Autodesk Fusion 360 part; units mm, degrees
(part 2 of 2)
  dimension "d115" = 6
  dimension "d116" = 6
  dimension "d117" = 6
  dimension "d118" = 6
  dimension "d119" = 6
  dimension "d120" = 6
  dimension "d121" = 6
  dimension "d122" = 6
  dimension "d123" = 6
  dimension "d124" = 6
  dimension "d125" = 6
  dimension "d126" = 6
  dimension "d195" = 0
  dimension "d196" = 40
  dimension "d199" = 0
  dimension "d200" = -133.5
  dimension "d203" = 240
  dimension "d204" = 0
  dimension "d207" = 0
  dimension "d208" = -240
  dimension "d211" = 0
  dimension "d212" = -133
  dimension "d215" = 0
  dimension "d216" = 40
  dimension "d219" = 0
  dimension "d220" = -269.838
  dimension "d223" = 0
  dimension "d224" = 269.838
  dimension "d225" = 200
  dimension "d226" = 330
  dimension "d227" = 40
  dimension "d228" = 40
  dimension "d229" = 40
  dimension "d230" = 40
  dimension "d231" = 60
  dimension "d232" = 90
  dimension "d233" = 90
  dimension "d234" = 110
  dimension "d235" = 110
  dimension "d236" = 110
  dimension "d237" = 120
  dimension "d238" = 55
  dimension "d239" = 55
  dimension "d240" = 55
  dimension "d241" = 55
  dimension "d242" = 16
  dimension "d243" = 25
  dimension "d244" = 25
  dimension "d245" = 35
  dimension "d246" = 12
  dimension "d247" = 19
  dimension "d248" = 50
  dimension "d249" = 5
  dimension "d250" = 150
  dimension "d251" = 22
  dimension "d252" = 22.5
  dimension "d253" = 22
  dimension "d254" = 6
  dimension "d255" = 200
  dimension "d256" = 269.3626
  dimension "d257" = 22
  dimension "d258" = 30
  dimension "d259" = 30
  dimension "d260" = 6
  dimension "d261" = 330
  dimension "d262" = 30
  dimension "d263" = 6
  dimension "d264" = 30
  dimension "d265" = 6
  dimension "d266" = 30
  dimension "d267" = 6
  dimension "d268" = 30
  dimension "d269" = 6
  dimension "d270" = 30
  dimension "d271" = 6
  dimension "d272" = 30
  dimension "d273" = 6
  dimension "d274" = 30
  dimension "d275" = 6
  dimension "d276" = 60
  dimension "d277" = 6
  dimension "d278" = 40
  dimension "d279" = 60
  dimension "d280" = 6
  dimension "d281" = 40
  dimension "d282" = 185.187
  dimension "d283" = 330
  dimension "d284" = 30
  dimension "d285" = 35
  dimension "d286" = 6
  dimension "d287" = 30
  dimension "d288" = 35
  dimension "d289" = 6
  dimension "d290" = 185.1872
  dimension "d291" = 185.187
  dimension "d292" = 30
  dimension "d293" = 30
  dimension "d294" = 6
  dimension "d295" = 35
  dimension "d296" = 15
  dimension "d297" = 10
  dimension "d298" = 6
  dimension "d299" = 35
  dimension "d300" = 330
  dimension "d301" = 20
  dimension "d302" = 17.5
  dimension "d303" = 6
  dimension "d304" = 6
  dimension "d305" = 6
  dimension "d306" = 6
  dimension "d307" = 6
  dimension "d308" = 6
  dimension "d309" = 6
  dimension "d310" = 6
  dimension "d311" = 6
  dimension "d312" = 6
  dimension "d313" = 6
  dimension "d314" = 6
  dimension "d315" = 6
  dimension "d316" = 6
  dimension "d317" = 6
  dimension "d318" = 6
  dimension "d319" = 6
  dimension "d320" = 6
  dimension "d321" = 6
  dimension "d322" = 6
  dimension "d323" = 6
  dimension "d324" = 6
  dimension "d325" = 6
  dimension "d326" = 6
  dimension "d327" = 6
  dimension "d328" = 6
  dimension "d329" = 6
  dimension "d330" = 6
  dimension "d331" = 300
  dimension "d332" = 35
  dimension "d333" = 5
  dimension "d334" = 150
  dimension "d335" = 20
  dimension "d336" = 200
  dimension "d337" = 269.3626
  dimension "d338" = 22
  dimension "d339" = 60
  dimension "d340" = 6
  dimension "d341" = 40
  dimension "d342" = 60
  dimension "d343" = 6
  dimension "d344" = 40
  dimension "d345" = 30
  dimension "d346" = 35
  dimension "d347" = 6
  dimension "d348" = 30
  dimension "d349" = 35
  dimension "d350" = 6
  dimension "d351" = 185.1872
  dimension "d352" = 35
  dimension "d353" = 15
  dimension "d354" = 10
  dimension "d355" = 6
  dimension "d356" = 6
  dimension "d357" = 6
  dimension "d358" = 6
  dimension "d359" = 6
  dimension "d360" = 6
  dimension "d361" = 6
  dimension "d362" = 6
  dimension "d363" = 6
  dimension "d364" = 6
  dimension "d365" = 6
  dimension "d366" = 6
  dimension "d367" = 5
  dimension "d368" = 20
  dimension "d369" = 5
  dimension "d370" = 6
  dimension "d371" = 5
  dimension "d372" = 9
  dimension "d373" = 20
  dimension "d374" = 9
  dimension "d375" = 5
  dimension "d376" = 9
  dimension "d377" = 9
  dimension "d378" = 9
  dimension "d379" = 9
  dimension "d380" = 9
  dimension "d381" = 9
  dimension "d382" = 9
  dimension "d383" = 9
  dimension "d384" = 9
  dimension "d385" = 9
  dimension "d386" = 9
  dimension "d387" = 6
  dimension "d388" = 15
  dimension "d389" = 6
  dimension "d390" = 15
  dimension "d391" = 6
  dimension "d392" = 15
  dimension "d393" = 6
  dimension "d394" = 15
  dimension "d395" = 6
  dimension "d396" = 15
  dimension "d397" = 6
  dimension "d398" = 15
  dimension "d399" = 6
  dimension "d400" = 5
  dimension "d401" = 9
  dimension "d402" = 20
  dimension "d403" = 9
  dimension "d404" = 5
  dimension "d405" = 6
  dimension "d406" = 6
  dimension "d407" = 5
  dimension "d408" = 9
  dimension "d409" = 20
  dimension "d410" = 9
  dimension "d411" = 5
  constraint vertical L19
  constraint horizontal L13
  constraint vertical L5
  constraint coincident L5.end L18.start
  constraint coincident L53.end L18
  constraint coincident L59.start L18
  constraint coincident L0.start L5
  constraint perpendicular L0 L5
  constraint horizontal L16
  constraint horizontal L11
  constraint horizontal L17
  constraint perpendicular L19 L56
  constraint perpendicular L19 L22
  constraint perpendicular L21 L56
  constraint perpendicular L19 L28
  constraint perpendicular L19 L61
  constraint perpendicular L24 L61
  constraint perpendicular L19 L20
  constraint perpendicular L19 L54
  constraint perpendicular L20 L52
  constraint perpendicular L27 L56
  constraint perpendicular L19 L30
  constraint perpendicular L18 L59
  constraint perpendicular L18 L23
  constraint perpendicular L18 L60
  constraint perpendicular L18 L36
  constraint perpendicular L14 L18
  constraint perpendicular L18 L42
  constraint perpendicular L18 L35
  constraint perpendicular L18 L39
  constraint perpendicular L18 L46
  constraint perpendicular L6 L18
  constraint perpendicular L5 L45
  constraint perpendicular L4 L5
  constraint perpendicular L4 L43
  constraint perpendicular L5 L51
  constraint perpendicular L5 L47
  constraint perpendicular L5 L37
  constraint horizontal L3
  constraint perpendicular L3 L8
  constraint perpendicular L11 L34
  constraint perpendicular L9 L11
  constraint perpendicular L31 L34
  constraint perpendicular L17 L32
  constraint perpendicular L1 L17
  constraint perpendicular L7 L32
  constraint perpendicular L11 L44
  constraint perpendicular L17 L48
  constraint perpendicular L44 L49
  constraint perpendicular L10 L13
  constraint perpendicular L11 L55
  constraint perpendicular L10 L15
  constraint perpendicular L17 L40
  constraint perpendicular L17 L25
  constraint perpendicular L40 L50
  constraint perpendicular L16 L58
  constraint perpendicular L17 L29
  constraint perpendicular L26 L58
  constraint vertical L81
  constraint horizontal L75
  constraint vertical L67
  constraint coincident L53.end L80
  constraint coincident L59.start L80
  constraint coincident L0.start L67
  constraint perpendicular L62 L67
  constraint horizontal L78
  constraint horizontal L73
  constraint horizontal L79
  constraint perpendicular L81 L118
  constraint perpendicular L81 L84
  constraint perpendicular L83 L118
  constraint perpendicular L81 L90
  constraint perpendicular L81 L123
  constraint perpendicular L86 L123
  constraint perpendicular L81 L82
  constraint perpendicular L81 L116
  constraint perpendicular L82 L114
  constraint perpendicular L89 L118
  constraint perpendicular L81 L92
  constraint perpendicular L80 L121
  constraint perpendicular L80 L85
  constraint perpendicular L80 L122
  constraint perpendicular L80 L98
  constraint perpendicular L76 L80
  constraint perpendicular L80 L104
  constraint perpendicular L80 L97
  constraint perpendicular L80 L101
  constraint perpendicular L80 L108
  constraint perpendicular L68 L80
  constraint perpendicular L67 L107
  constraint perpendicular L66 L67
  constraint perpendicular L66 L105
  constraint perpendicular L67 L113
  constraint perpendicular L67 L109
  constraint perpendicular L67 L99
  constraint horizontal L65
  constraint perpendicular L65 L70
  constraint perpendicular L73 L96
  constraint perpendicular L71 L73
  constraint perpendicular L93 L96
  constraint perpendicular L79 L94
  constraint perpendicular L63 L79
  constraint perpendicular L69 L94
  constraint perpendicular L73 L106
  constraint perpendicular L79 L110
  constraint perpendicular L106 L111
  constraint perpendicular L72 L75
  constraint perpendicular L73 L117
  constraint perpendicular L72 L77
  constraint perpendicular L79 L102
  constraint perpendicular L79 L87
  constraint perpendicular L102 L112
  constraint perpendicular L78 L120
  constraint perpendicular L79 L91
  constraint perpendicular L88 L120
  constraint vertical L143
  constraint horizontal L137
  constraint vertical L129
  constraint coincident L53.end L142
  constraint coincident L59.start L142
  constraint coincident L0.start L129
  constraint perpendicular L124 L129
  constraint horizontal L140
  constraint horizontal L135
  constraint horizontal L141
  constraint perpendicular L143 L180
  constraint perpendicular L143 L146
  constraint perpendicular L145 L180
  constraint perpendicular L143 L152
  constraint perpendicular L143 L185
  constraint perpendicular L148 L185
  constraint perpendicular L143 L144
  constraint perpendicular L143 L178
  constraint perpendicular L144 L176
  constraint perpendicular L151 L180
  constraint perpendicular L143 L154
  constraint perpendicular L142 L183
  constraint perpendicular L142 L147
  constraint perpendicular L142 L184
  constraint perpendicular L142 L160
  constraint perpendicular L138 L142
  constraint perpendicular L142 L166
  constraint perpendicular L142 L159
  constraint perpendicular L142 L163
  constraint perpendicular L142 L170
  constraint perpendicular L130 L142
  constraint perpendicular L129 L169
  constraint perpendicular L128 L129
  constraint perpendicular L128 L167
  constraint perpendicular L129 L175
  constraint perpendicular L129 L171
  constraint perpendicular L129 L161
  constraint horizontal L127
  constraint perpendicular L127 L132
  constraint perpendicular L135 L158
  constraint perpendicular L133 L135
  constraint perpendicular L155 L158
  constraint perpendicular L141 L156
  constraint perpendicular L125 L141
  constraint perpendicular L131 L156
  constraint perpendicular L135 L168
  constraint perpendicular L141 L172
  constraint perpendicular L168 L173
  constraint perpendicular L134 L137
  constraint perpendicular L135 L179
  constraint perpendicular L134 L139
  constraint perpendicular L141 L164
  constraint perpendicular L141 L149
  constraint perpendicular L164 L174
  constraint perpendicular L140 L182
  constraint perpendicular L141 L153
  constraint perpendicular L150 L182
  constraint perpendicular L315 L588
  constraint horizontal L348
  constraint vertical L466
  constraint perpendicular L190 L499
  constraint horizontal L231
  constraint vertical L386
  constraint horizontal L197
  constraint vertical L551
  constraint horizontal L337
  constraint vertical L254
  constraint horizontal L366
  constraint vertical L585
  constraint coincident L240.end L564
  constraint coincident L204.start L564
  constraint perpendicular L204 L564
  constraint perpendicular L204 L281
  constraint coincident L205.end L564
  constraint perpendicular L205 L564
  constraint coincident L528.start L588
  constraint coincident L568.start L588
  constraint coincident L583.end L588
  constraint coincident L548.start L588
  constraint coincident L343.start L588
  constraint coincident L339.start L588
  constraint coincident L372.start L588
  constraint coincident L325.start L588
  constraint coincident L558.start L588
  constraint coincident L305.start L523
  constraint perpendicular L523 L541
  constraint perpendicular L296 L541
  constraint coincident P228 L523
  constraint perpendicular L358 L523
  constraint coincident L305.start L360
  constraint perpendicular L333 L360
  constraint perpendicular L333 L335
  constraint coincident P228 L360
  constraint perpendicular L360 L538
  constraint perpendicular L304 L553
  constraint perpendicular L347 L351
  constraint perpendicular L341 L580
  constraint perpendicular L305 L342
  constraint perpendicular L572 L576
  constraint perpendicular L376 L595
  constraint coincident L293.start L315
  constraint perpendicular L293 L315
  constraint perpendicular L293 L329
  constraint coincident L357.end L315
  constraint perpendicular L315 L357
  constraint coincident L569.start L315
  constraint perpendicular L315 L569
  constraint perpendicular L525 L569
  constraint coincident L350.end L315
  constraint perpendicular L315 L350
  constraint horizontal L447
  constraint horizontal L330
  constraint vertical L298
  constraint coincident L533.start L540
  constraint perpendicular L533 L540
  constraint perpendicular L364 L533
  constraint coincident L290.end L540
  constraint perpendicular L290 L540
  constraint perpendicular L314 L540
  constraint perpendicular L314 L584
  constraint coincident L375.end L540
  constraint coincident L612.start L447
  constraint coincident L322.start L447
  constraint horizontal L459
  constraint coincident L291.start L459
  constraint coincident L300.start L459
  constraint coincident L319.start L298
  constraint perpendicular L298 L319
  constraint perpendicular L308 L319
  constraint coincident P107 L298
  constraint perpendicular L298 L332
  constraint coincident L556.start L190
  constraint perpendicular L190 L556
  constraint perpendicular L246 L556
  constraint coincident L409.end L190
  constraint perpendicular L190 L409
  constraint vertical L475
  constraint horizontal L486
  constraint vertical L509
  constraint coincident L314.start L498
  constraint coincident L227.start L250
  constraint coincident L384.start L250
  constraint coincident L251.start L486
  constraint coincident L429.start L486
  constraint perpendicular L558 L588
  constraint perpendicular L318 L588
  constraint perpendicular L372 L588
  constraint perpendicular L339 L588
  constraint perpendicular L343 L588
  constraint perpendicular L548 L588
  constraint perpendicular L568 L588
  constraint perpendicular L528 L588
  constraint perpendicular L369 L588
  constraint perpendicular L289 L459
  constraint perpendicular L291 L459
  constraint perpendicular L300 L447
  constraint perpendicular L322 L447
  constraint perpendicular L300 L301
  constraint perpendicular L447 L612
  constraint perpendicular L459 L590
  constraint perpendicular L542 L612
  constraint perpendicular L330 L352
  constraint perpendicular L320 L355
  constraint perpendicular L320 L549
  constraint perpendicular L317 L522
  constraint perpendicular L317 L455
  constraint perpendicular L320 L610
  constraint perpendicular L373 L455
  constraint perpendicular L346 L549
  constraint perpendicular L352 L361
  constraint perpendicular L227 L250
  constraint perpendicular L250 L412
  constraint perpendicular L250 L384
  constraint perpendicular L250 L401
  constraint perpendicular L486 L501
  constraint perpendicular L251 L486
  constraint perpendicular L429 L486
  constraint perpendicular L266 L486
  constraint perpendicular L316 L555
  constraint perpendicular L313 L577
  constraint horizontal L566
  constraint vertical L559
  constraint horizontal L483
  constraint vertical L452
  constraint coincident L268.start L555
  constraint coincident L252.start L555
  constraint coincident L437.end L555
  constraint coincident L407.start L555
  constraint coincident L402.start L555
  constraint coincident L229.start L555
  constraint coincident L394.start L555
  constraint coincident L421.start L555
  constraint coincident L613.start L555
  constraint coincident L387.start L316
  constraint perpendicular L316 L387
  constraint perpendicular L189 L387
  constraint coincident L245.end L316
  constraint perpendicular L245 L316
  constraint coincident L440.start L316
  constraint perpendicular L316 L440
  constraint perpendicular L440 L602
  constraint coincident L428.end L316
  constraint perpendicular L316 L428
  constraint coincident L457.start L560
  constraint perpendicular L457 L560
  constraint perpendicular L457 L615
  constraint coincident L453.end L560
  constraint perpendicular L453 L560
  constraint perpendicular L380 L560
  constraint perpendicular L380 L531
  constraint coincident L345.end L560
  constraint perpendicular L345 L560
  constraint coincident L446.start L577
  constraint perpendicular L446 L577
  constraint perpendicular L446 L605
  constraint coincident L599.end L577
  constraint perpendicular L577 L599
  constraint coincident L380.start L537
  constraint perpendicular L555 L613
  constraint perpendicular L489 L555
  constraint perpendicular L394 L555
  constraint perpendicular L229 L555
  constraint perpendicular L402 L555
  constraint perpendicular L407 L555
  constraint perpendicular L252 L555
  constraint perpendicular L268 L555
  constraint perpendicular L288 L555
  constraint perpendicular L312 L370
  constraint perpendicular L370 L500
  constraint perpendicular L206 L500
  constraint perpendicular L238 L510
  constraint perpendicular L313 L477
  constraint perpendicular L477 L594
  constraint perpendicular L425 L594
  constraint perpendicular L425 L607
  constraint perpendicular L454 L607
  constraint perpendicular L454 L488
  constraint coincident L481.end L313
  constraint perpendicular L313 L481
  constraint perpendicular L206 L422
  constraint perpendicular L397 L515
  constraint perpendicular L435 L484
  constraint perpendicular L545 L591
  constraint perpendicular L438 L575
  constraint perpendicular L521 L589
  constraint perpendicular L238 L465
  constraint perpendicular L444 L499
  constraint perpendicular L460 L498
  constraint perpendicular L470 L499
  constraint perpendicular L470 L517
  constraint perpendicular L507 L517
  constraint perpendicular L507 L608
  constraint perpendicular L499 L520
  constraint perpendicular L399 L499
  constraint perpendicular L191 L399
  constraint perpendicular L191 L417
  constraint perpendicular L224 L417
  constraint perpendicular L224 L416
  constraint perpendicular L416 L423
  constraint coincident L215.end L499
  constraint perpendicular L215 L499
  constraint coincident L596.end L312
  constraint perpendicular L312 L596
  constraint coincident L546.end L312
  constraint perpendicular L312 L546
  constraint coincident L611.end L312
  constraint perpendicular L312 L611
  constraint coincident L519.end L312
  constraint perpendicular L312 L519
  constraint coincident L408.end L312
  constraint perpendicular L312 L408
  constraint coincident L382.end L313
  constraint perpendicular L313 L382
  measures "d1" distance of L5.end L3.start
  measures "d2" distance of L5.end L18.end
  measures "d3" diameter of A0
  measures "d4" distance of A0.centre L5
  measures "d5" distance of A0.centre L19
  measures "d6" distance of L0.end L0.start
  measures "d7" distance of L21.end L18.end
  measures "d8" distance of L21.start L22.start
  measures "d9" distance of L24.end L28.start
  measures "d10" distance of L24.start L61.start
  measures "d11" distance of L20.end L20.start
  measures "d12" distance of L52.start P11
  measures "d13" distance of L27.end L18.end
  measures "d14" distance of L27.end L30.end
  measures "d15" distance of L57.end L59.start
  measures "d16" distance of L23.end L23.start
  measures "d17" distance of L12.end L60.start
  measures "d18" distance of L12.start L36.start
  measures "d19" distance of L14.end L14.start
  measures "d20" distance of L41.start L42.start
  measures "d21" distance of L33.end L35.start
  measures "d22" distance of L33.start L39.start
  measures "d23" distance of L2.end L5.end
  measures "d24" distance of L2.start L6.start
  measures "d25" distance of L43.end L5.end
  measures "d26" distance of L4.end L4.start
  measures "d27" distance of L38.end L51.start
  measures "d28" distance of L38.start L47.start
  measures "d29" distance of L8.end L37.start
  measures "d30" distance of L3.end L3.start
  measures "d31" distance of L31.end L3.start
  measures "d32" distance of L9.end L9.start
  measures "d33" distance of L7.end L32.start
  measures "d34" distance of L1.end L1.start
  measures "d35" distance of L44.end L44.start
  measures "d36" distance of L48.end L48.start
  measures "d37" distance of L10.end L10.start
  measures "d38" distance of L15.start L55.start
  measures "d39" distance of L40.end L40.start
  measures "d40" distance of L25.end L25.start
  measures "d41" distance of L26.end L58.start
  measures "d42" distance of L26.start P11
  measures "d43" distance of L5.end L3.start
  measures "d44" distance of L5.end L18.end
  measures "d45" diameter of A1
  measures "d46" distance of A0.centre L67
  measures "d47" distance of A0.centre L81
  measures "d48" distance of L0.end L0.start
  measures "d49" distance of L21.end L18.end
  measures "d50" distance of L21.start L22.start
  measures "d51" distance of L24.end L28.start
  measures "d52" distance of L24.start L61.start
  measures "d53" distance of L20.end L20.start
  measures "d54" distance of L52.start P11
  measures "d55" distance of L27.end L18.end
  measures "d56" distance of L27.end L30.end
  measures "d57" distance of L57.end L59.start
  measures "d58" distance of L23.end L23.start
  measures "d59" distance of L12.end L60.start
  measures "d60" distance of L12.start L36.start
  measures "d61" distance of L14.end L14.start
  measures "d62" distance of L41.start L42.start
  measures "d63" distance of L33.end L35.start
  measures "d64" distance of L33.start L39.start
  measures "d65" distance of L2.end L5.end
  measures "d66" distance of L2.start L6.start
  measures "d67" distance of L43.end L5.end
  measures "d68" distance of L4.end L4.start
  measures "d69" distance of L38.end L51.start
  measures "d70" distance of L38.start L47.start
  measures "d71" distance of L8.end L37.start
  measures "d72" distance of L3.end L3.start
  measures "d73" distance of L31.end L3.start
  measures "d74" distance of L9.end L9.start
  measures "d75" distance of L7.end L32.start
  measures "d76" distance of L1.end L1.start
  measures "d77" distance of L44.end L44.start
  measures "d78" distance of L48.end L48.start
  measures "d79" distance of L10.end L10.start
  measures "d80" distance of L15.start L55.start
  measures "d81" distance of L40.end L40.start
  measures "d82" distance of L25.end L25.start
  measures "d83" distance of L26.end L58.start
  measures "d84" distance of L26.start P11
  measures "d85" distance of L5.end L3.start
  measures "d86" distance of L5.end L18.end
  measures "d87" diameter of A2
  measures "d88" distance of A0.centre L129
  measures "d89" distance of A0.centre L143
  measures "d90" distance of L0.end L0.start
  measures "d91" distance of L21.end L18.end
  measures "d92" distance of L21.start L22.start
  measures "d93" distance of L24.end L28.start
  measures "d94" distance of L24.start L61.start
  measures "d95" distance of L20.end L20.start
  measures "d96" distance of L52.start P11
  measures "d97" distance of L27.end L18.end
  measures "d98" distance of L27.end L30.end
  measures "d99" distance of L57.end L59.start
  measures "d100" distance of L23.end L23.start
  measures "d101" distance of L12.end L60.start
  measures "d102" distance of L12.start L36.start
  measures "d103" distance of L14.end L14.start
  measures "d104" distance of L41.start L42.start
  measures "d105" distance of L33.end L35.start
  measures "d106" distance of L33.start L39.start
  measures "d107" distance of L2.end L5.end
  measures "d108" distance of L2.start L6.start
  measures "d109" distance of L43.end L5.end
  measures "d110" distance of L4.end L4.start
  measures "d111" distance of L38.end L51.start
  measures "d112" distance of L38.start L47.start
  measures "d113" distance of L8.end L37.start
  measures "d114" distance of L3.end L3.start
  measures "d115" distance of L31.end L3.start
  measures "d116" distance of L9.end L9.start
  measures "d117" distance of L7.end L32.start
  measures "d118" distance of L1.end L1.start
  measures "d119" distance of L44.end L44.start
  measures "d120" distance of L48.end L48.start
  measures "d121" distance of L10.end L10.start
  measures "d122" distance of L15.start L55.start
  measures "d123" distance of L40.end L40.start
  measures "d124" distance of L25.end L25.start
  measures "d125" distance of L26.end L58.start
  measures "d126" distance of L26.start P11
  measures "d225" distance of L360.end L240.start
  measures "d226" distance of L360.start L360.end
  measures "d227" diameter of A3
  measures "d228" diameter of A5
  measures "d229" diameter of A6
  measures "d230" diameter of A7
  measures "d231" distance of A3.centre L348
  measures "d232" distance of A6.centre L348
  measures "d233" distance of A7.centre L348
  measures "d234" distance of A6.centre A7.centre
  measures "d235" distance of A6.centre L564
  measures "d236" distance of A7.centre L466
  measures "d237" distance of A5.centre L348
  measures "d238" horizontal distance of A6.centre A3.centre
  measures "d239" horizontal distance of A7.centre A3.centre
  measures "d240" horizontal distance of A6.centre A5.centre
  measures "d241" horizontal distance of A7.centre A5.centre
  measures "d242" diameter of A4
  measures "d243" distance of A4.centre L348
  measures "d244" distance of A4.centre L564
  measures "d245" distance of L190.end L190.start
  measures "d246" distance of L231.end L231.start
  measures "d247" distance of L231.end L197.start
  measures "d248" distance of L190 L231
  measures "d249" distance of L366.end L337.start
  measures "d250" distance of L254.start L337.start
  measures "d251" distance of L204 L348
  measures "d252" distance of L204.end L205.start
  measures "d253" distance of L205 L263
  measures "d254" distance of L204.start L204.end
  measures "d255" distance of L315.start L190.start
  measures "d256" distance of L315.start L315.end
  measures "d257" distance of L558.start L190.start
  measures "d258" distance of L541 L564
  measures "d259" distance of L296.end L296.start
  measures "d260" distance of L305.start L296.start
  measures "d261" distance of L360.end L360.start
  measures "d262" distance of L296.end L296.start
  measures "d263" distance of L296.start L305.start
  measures "d264" distance of L296.end L296.start
  measures "d265" distance of L296.start L305.start
  measures "d266" distance of L296.start L296.end
  measures "d267" distance of L296.start L305.start
  measures "d268" distance of L296.start L296.end
  measures "d269" distance of L296.start L305.start
  measures "d270" distance of L296.end L296.start
  measures "d271" distance of L296.start L305.start
  measures "d272" distance of L296.end L296.start
  measures "d273" distance of L305.start L296.start
  measures "d274" distance of L296.start L296.end
  measures "d275" distance of L305.start L296.start
  measures "d276" distance of L293 L588
  measures "d277" distance of L293.end L293.start
  measures "d278" distance of L293.end L329.end
  measures "d279" distance of L315.end L569
  measures "d280" distance of L350.end L350.start
  measures "d281" distance of L350.start L525.start
  measures "d282" distance of L289.start L312.start
  measures "d283" distance of L312.end L312.start
  measures "d284" distance of L315.end L533
  measures "d285" distance of L290.start L364.start
  measures "d286" distance of L290.end L290.start
  measures "d287" distance of L444.start L314
  measures "d288" distance of L375.start L314.end
  measures "d289" distance of L375.start L375.end
  measures "d290" distance of L315.end L499
  measures "d291" distance of L312.start L289.start
  measures "d292" distance of L319 L447
  measures "d293" distance of L308.start L308.end
  measures "d294" distance of L319.start L308.start
  measures "d295" distance of L190.end L190.start
  measures "d296" distance of L246.end L246.start
  measures "d297" distance of L190.start L556
  measures "d298" distance of L246.end L409.end
  measures "d299" distance of L250.start L250.end
  measures "d300" distance of L250.end L266.start
  measures "d301" diameter of A8
  measures "d302" distance of A8.centre L509
  measures "d303" distance of L307.start L558.start
  measures "d304" distance of L307.end L190.start
  measures "d305" distance of L325.start L325.end
  measures "d306" distance of L372.start L372.end
  measures "d307" distance of L339.end L339.start
  measures "d308" distance of L343.start L343.end
  measures "d309" distance of L548.start L334.end
  measures "d310" distance of L568.start L334.start
  measures "d311" distance of L528.start L323.end
  measures "d312" distance of L315.start L323.start
  measures "d313" distance of L289.start L289.end
  measures "d314" distance of L291.start L291.end
  measures "d315" distance of L322.start L301.start
  measures "d316" distance of L612.start L542.end
  measures "d317" distance of L352.end L298.start
  measures "d318" distance of L355.start L355.end
  measures "d319" distance of L549.start L346.end
  measures "d320" distance of L346.start L522.start
  measures "d321" distance of L373.end L455.start
  measures "d322" distance of L312.end L373.start
  measures "d323" distance of L227.start L186.start
  measures "d324" distance of L250.start L186.end
  measures "d325" distance of L384.end L384.start
  measures "d326" distance of L250.end L401.end
  measures "d327" distance of L486.end L474.end
  measures "d328" distance of L251.start L251.end
  measures "d329" distance of L429.end L429.start
  measures "d330" distance of L266.end L266.start
  measures "d331" distance of L537.end L437.start
  measures "d332" distance of L313.start L437.start
  measures "d333" distance of L452.end L452.start
  measures "d334" distance of L452.end L559.start
  measures "d335" distance of L313 L559
  measures "d336" distance of L288.start L437.start
  measures "d337" distance of L316.end L288.start
  measures "d338" distance of L613.start L437.start
  measures "d339" distance of L387 L555
  measures "d340" distance of L387.start L189.start
  measures "d341" distance of L189.end L189.start
  measures "d342" distance of L316.end L440
  measures "d343" distance of L428.start L428.end
  measures "d344" distance of L428.start L440.end
  measures "d345" distance of L316.end L457
  measures "d346" distance of L457.end L453.start
  measures "d347" distance of L453.end L453.start
  measures "d348" distance of L313.end L380
  measures "d349" distance of L380.end L345.start
  measures "d350" distance of L345.end L345.start
  measures "d351" distance of L316.end L313
  measures "d352" distance of L313.start L437.start
  measures "d353" distance of L599.start L446.end
  measures "d354" distance of L437.start L446
  measures "d355" distance of L599.start L599.end
  measures "d356" distance of L613.start L495.start
  measures "d357" distance of L437.start L489.end
  measures "d358" distance of L421.start L212.end
  measures "d359" distance of L212.start L394.start
  measures "d360" distance of L229.start L229.end
  measures "d361" distance of L402.start L402.end
  measures "d362" distance of L407.start L193.end
  measures "d363" distance of L252.start L193.start
  measures "d364" distance of L268.start L268.end
  measures "d365" distance of L288.start L282.start
  measures "d366" distance of L370.end L317.end
  measures "d367" distance of L206.start L370.end
  measures "d368" distance of L206.end L422.start
  measures "d369" distance of L238.end L238.start
  measures "d370" distance of L477.end L313.start
  measures "d371" distance of L477.end L425.start
  measures "d372" distance of L425.end L425.start
  measures "d373" distance of L425.end L454.start
  measures "d374" distance of L454.end L454.start
  measures "d375" distance of L454.end L481.start
  measures "d376" distance of L238.start L422.start
  measures "d377" distance of L397.start L397.end
  measures "d378" distance of L418.start L371.start
  measures "d379" distance of L270.start L202.start
  measures "d380" distance of L257.end L435.end
  measures "d381" distance of L441.start L441.end
  measures "d382" distance of L545.start L545.end
  measures "d383" distance of L374.end L374.start
  measures "d384" distance of L438.start L438.end
  measures "d385" distance of L529.start L378.start
  measures "d386" distance of L521.end L521.start
  measures "d387" distance of L242.end L242.start
  measures "d388" distance of L312 L515
  measures "d389" distance of L238.end L465.end
  measures "d390" distance of L312 L422
  measures "d391" distance of L283.start L257.start
  measures "d392" distance of L312 L484
  measures "d393" distance of L532.start L532.end
  measures "d394" distance of L312 L591
  measures "d395" distance of L579.start L579.end
  measures "d396" distance of L312 L575
  measures "d397" distance of L432.start L432.end
  measures "d398" distance of L312 L589
  measures "d399" distance of L444.end L444.start
  measures "d400" distance of L444.end L460.end
  measures "d401" distance of L470.end L460.end
  measures "d402" distance of L470.end L507.start
  measures "d403" distance of L507.end L507.start
  measures "d404" distance of L507.end L520.start
  measures "d405" distance of L520.end L520.start
  measures "d406" distance of L191.start L190.end
  measures "d407" distance of L191.start L191.end
  measures "d408" distance of L224.start L191.end
  measures "d409" distance of L224.end L224.start
  measures "d410" distance of L416.end L224.end
  measures "d411" distance of L416.end L215.start
extrude "Extrude1" add sketch "Sketch1" along normal blind 6 makes body 1 at (0, -1201.8379, 340.7175) makes body 2 at (0, -1095.8388, 89.5085) makes body 3 at (0, -1660.57, -146.8734) makes body 4 at (0, -1303.6898, 85.5978) makes body 5 at (0, -1282.3066, -237.6856) makes body 6 at (0, -1717.643, 453.3188)
